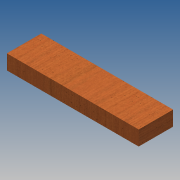
# Autodesk Inventor part: 2p3ph
Saved by Autodesk Inventor 2014 SP1 (Build 180222100, 222)
## iProperties
Company: HERA Project
Created: 2013-09-06
Part Number: 2p3ph
Material: Wood (Cherry)
Document SubType Name: Modeling
Designer: David DeBoer
Density: 0.5 g/cm^3
Mass: 635.373 g
Surface Area: 1042.45 cm^2
Volume: 1270.75 cm^3
Description: post horizontal holder
Appearance: Cherry - Natural Low Gloss
Author: David DeBoer
Autodesk Inventor part; units mm, degrees
ref_plane "YZ Plane" through (0, 0, 0) normal (1, 0, 0) x (0, 1, 0)
ref_plane "XZ Plane" through (0, 0, 0) normal (0, 1, 0) x (-1, 0, 0)
ref_plane "XY Plane" through (0, 0, 0) normal (0, 0, 1) x (1, 0, 0)
sketch "Sketch1" plane through (0, 0, 0) normal (0, 0, 1) x (1, 0, 0)
  line L0 (0, 0) -> (340.36, 0)
  line L1 (0, 0) -> (0, 38.1)
  line L2 (0, 38.1) -> (340.36, 38.1)
  line L3 (340.36, 0) -> (340.36, 38.1)
  dimension "d0" = 340.36
  dimension "d1" = 38.1
  dimension "d2" = 90
  constraints: 8 end point, 2 perpendicular
  measures "d0" distance of L0.start L0.end
  measures "d1" distance of L0.start L1.end
  measures "d2" angle of L3 L0
extrude "Extrusion1" add sketch "Sketch1" along normal blind 88.9
body "Solid1"
